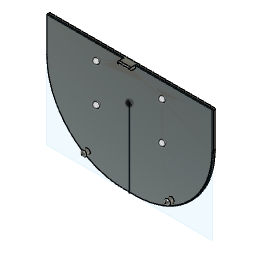
2ndfinal trayholder updated v3 (Autodesk Fusion 360 design; units mm, degrees)
Autodesk Fusion 360 part; units mm, degrees
note: some values were not read from the file. Chosen so that the rebuilt part matches the saved one: which pieces of a blend or face edit are solid.
sketch "Sketch1" plane through (0, 0, 0) normal (0, 1, 0) x (1, 0, 0)
  line L0 (139, 95) -> (-139, 95)
  line L1 (-139, 95) -> (-139, -95)
  line L2 (-139, -95) -> (139, -95)
  line L3 (139, -95) -> (139, 95)
  line L4 (139, 95) -> (-139, -95) construction
  line L5 (-139, 95) -> (139, -95) construction
  dimension "d1" = 278
  dimension "d2" = 190
  constraint horizontal L0
  constraint perpendicular L0 L1
  constraint parallel L0 L2
  constraint parallel L1 L3
  constraint coincident L4 origin
  constraint coincident L5 origin
  measures "d1" distance of L1.end L2.end
  measures "d2" distance of L0.end L1.end
extrude "Extrude1" add sketch "Sketch1" along normal blind 5
sketch "Sketch2" plane through (0, 0, 0) normal (0, -1, 0) x (1, 0, 0)
  line L0 (139, -95) -> (139, 95)
  line L1 (139, 95) -> (-139, 95)
  line L2 (-139, 95) -> (-139, -95)
  line L3 (-139, -95) -> (139, -95)
  line L4 (0, -95) -> (0, 35)
  dimension "d5" = 130
  dimension "d16" = 60
  constraint midpoint L3 L4.start
  constraint perpendicular L3 L4
  measures "d5" distance of L4.start L4.end
  measures "d16" distance of L1 L4.end
fillet "Fillet1" radius 130 2 edges at (-139, 2.5, -95) (139, 2.5, -95)
sketch "Sketch3" plane through (0, 0, 0) normal (0, -1, 0) x (1, 0, 0)
  arc A0 (9, -95) -> (139, 35) centre (9, 35) ccw
  line L0 (139, 35) -> (139, 95)
  line L1 (139, 95) -> (-139, 95)
  line L2 (-139, 95) -> (-139, 35)
  arc A1 (-139, 35) -> (-9, -95) centre (-9, 35) ccw
  line L3 (-9, -95) -> (9, -95)
  circle A2 centre (-70, -70) radius 4.5
  line L4 (0, 0) -> (0, -102.7377)
  circle A3 centre (70, -70) radius 4.5
  dimension "d21" = 9
  dimension "d24" = 140
  constraint coincident L4.start origin
  constraint vertical L4
  constraint symmetric A2 L4 A3
  measures "d21" diameter of A2
  measures "d24" distance of A2.centre A3.centre
extrude "Extrude3" add sketch "Sketch3" along normal blind 10 contours A2 | A3
fillet "Fillet2" radius 4 2 edges at (-74.1955, -10, -71.6273) (65.8045, -10, -71.6273)
sketch "Sketch4" plane through (0, 0, 0) normal (0, -1, 0) x (1, 0, 0)
  circle A0 centre (70, -70) radius 4.5
  circle A1 centre (-70, -70) radius 4.5
  arc A2 (9, -95) -> (139, 35) centre (9, 35) ccw
  line L0 (139, 35) -> (139, 95)
  line L1 (139, 95) -> (-139, 95)
  line L2 (-139, 95) -> (-139, 35)
  arc A3 (-139, 35) -> (-9, -95) centre (-9, 35) ccw
  line L3 (-9, -95) -> (9, -95)
  line L4 (-10, 95) -> (10, 95)
  line L5 (10, 95) -> (10, 90)
  line L6 (10, 90) -> (-10, 90)
  line L7 (-10, 90) -> (-10, 95)
  dimension "d29" = 5
  constraint horizontal L4
  constraint vertical L5
  constraint horizontal L6
  constraint vertical L7
  constraint coincident L1 L4.start
  measures "d29" distance of L4.start L6.end
extrude "Extrude4" add sketch "Sketch4" along normal blind 10 contours L1 L4 L5 L6 L7
fillet "Fillet3" radius 4 2 edges at (0, -10, 90) (0, -10, 95)
sketch "Sketch5" plane through (0, 0, 0) normal (0, -1, 0) x (1, 0, 0)
  point P0 (-55, 68.5)
  point P1 (55, 68.5)
  point P2 (55, 5)
  point P3 (-55, 5)
hole "Hole4" at (-55, 0, 68.5) at (-55, 0, 5) at (55, 0, 5) at (55, 0, 68.5) direction (0, 1, 0) diameter 5 depth 5 tip angle 180 counterbore diameter 9 counterbore depth 2.5
fillet "Fillet4" radius 2 2 edges at (139, 2.5, 95) (-139, 2.5, 95)
fillet "Fillet5" radius 1 17 edges at (138.4142, 5, 94.4142) (139, 5, 64) (100.9239, 5, -56.9239) (0, 5, -95) (-100.9239, 5, -56.9239) (-139, 5, 64) (-138.4142, 5, 94.4142) (0, 5, 95) (73.5, 0, 95) (138.4142, 0, 94.4142) (139, 0, 64) (100.9239, 0, -56.9239) (0, 0, -95) (-100.9239, 0, -56.9239) (-139, 0, 64) (-138.4142, 0, 94.4142) (-73.5, 0, 95)
